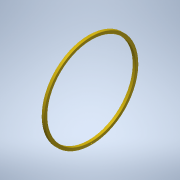
# Autodesk Inventor part: Kolo R600
Saved by Autodesk Inventor 2021 (Build 250183000, 183)
## iProperties
Created: 2024-04-08
Part Number: Kolo R600
Material: Steel
Document SubType Name: Modeling
Designer: Michal
Density: 7.85 g/cm^3
Appearance: Glossy - Gold
Author: Michal
Autodesk Inventor part; units mm, degrees
ref_plane "YZ Plane" through (0, 0, 0) normal (1, 0, 0) x (0, 1, 0)
ref_plane "XZ Plane" through (0, 0, 0) normal (0, 1, 0) x (-1, 0, 0)
ref_plane "XY Plane" through (0, 0, 0) normal (0, 0, 1) x (1, 0, 0)
sketch "Sketch1" plane through (0, 0, 0) normal (0, 1, 0) x (-1, 0, 0)
  line L0 (-7, 9) -> (7, 9) construction
  line L1 (9, 7) -> (9, -7) construction
  line L2 (7, -9) -> (-7, -9) construction
  line L3 (-9, -7) -> (-9, 7) construction
  line L4 (-9, 9) -> (9, -9) construction
  line L5 (9, 9) -> (-9, -9) construction
  arc A0 (9, 7) -> (7, 9) centre (7, 7) ccw construction
  arc A1 (7, -9) -> (9, -7) centre (7, -7) ccw construction
  arc A2 (-9, -7) -> (-7, -9) centre (-7, -7) ccw construction
  arc A3 (-7, 9) -> (-9, 7) centre (-7, 7) ccw construction
  line L6 (-7, -10) -> (7, -10)
  arc A4 (7, -10) -> (10, -7) centre (7, -7) ccw
  line L7 (10, -7) -> (10, 7)
  arc A5 (10, 7) -> (7, 10) centre (7, 7) ccw
  line L8 (7, 10) -> (-7, 10)
  arc A6 (-7, 10) -> (-10, 7) centre (-7, 7) ccw
  line L9 (-10, 7) -> (-10, -7)
  arc A7 (-10, -7) -> (-7, -10) centre (-7, -7) ccw
  line L10 (8, -7) -> (8, 7)
  arc A8 (8, 7) -> (7, 8) centre (7, 7) ccw
  line L11 (7, 8) -> (-7, 8)
  arc A9 (-7, 8) -> (-8, 7) centre (-7, 7) ccw
  line L12 (-8, 7) -> (-8, -7)
  arc A10 (-8, -7) -> (-7, -8) centre (-7, -7) ccw
  line L13 (-7, -8) -> (7, -8)
  arc A11 (7, -8) -> (8, -7) centre (7, -7) ccw
  point P0 (0, 0)
  point P1 (0, 0)
  point P2 (0, 0)
  dimension "d10" = 2
  dimension "depth" = 20
  dimension "width" = 20
  dimension "thickness" = 2
  constraints: 28 end point, 24 point on circle, 12 centre point, 8 point on line, 8 tangent, 6 parallel, 3 equal radius, 3 midpoint, 3 perpendicular, 1 coincident, 1 horizontal, 15 other
  measures "d10" radius of A0
  measures "depth" distance between parallel lines of L6 L8
  measures "width" distance between parallel lines of L9 L7
  measures "thickness" distance between parallel lines of L10 L7
sketch "Sketch3" plane through (0, 0, 0) normal (1, 0, 0) x (0, 1, 0)
  line L0 (-420, 0) -> (420, 0) projected
  circle A0 centre (0, 300) radius 300
  line L1 (0, -120) -> (0, 720) projected
  point P0 (0, 0)
  dimension "d62" = 600
  constraints: 1 centre point, 1 midpoint, 1 tangent
  measures "d62" diameter of A0
sweep "Sweep1" add profiles "Sketch1" path "Sketch3" path curves A0
sketch "Sketch6" plane through (10, 0, 300) normal (1, 0, 0) x (0, 0, -1)
  point P0 (300, 0)
  point P1 (300, 0)
  constraints: 1 coincident
hole "Hole4" at (10, 0, 0) direction (-1, 0, 0) diameter 6 end through all
equation "\"d10\" = thickness"
body "Solid2"
